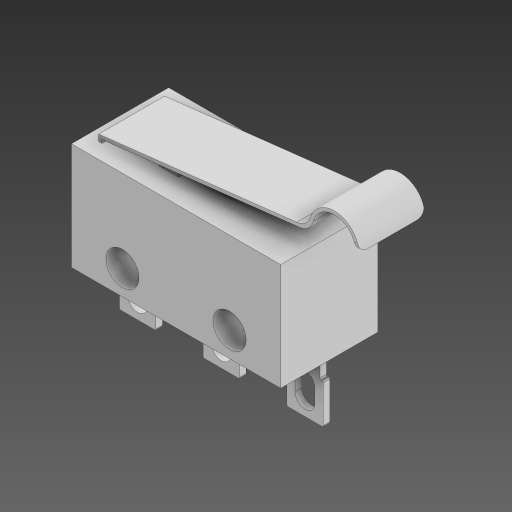
# Autodesk Inventor part: SS0750302F035S1A (Limit Switch)
Saved by Autodesk Inventor 2024 (Build 280153000, 153)
## iProperties
Created: 2024-02-03
Part Number: SS0750302F035S1A (Limit Switch)
Material: Generic
Document SubType Name: Modeling
Designer: david
Density: 1 g/cm^3
Appearance: Default
Author: david
Autodesk Inventor part; units mm, degrees
ref_plane "YZ Plane" through (0, 0, 0) normal (1, 0, 0) x (0, 1, 0)
ref_plane "XZ Plane" through (0, 0, 0) normal (0, 1, 0) x (-1, 0, 0)
ref_plane "XY Plane" through (0, 0, 0) normal (0, 0, 1) x (1, 0, 0)
sketch "Sketch1" plane through (0, 0, 0) normal (0, 0, 1) x (1, 0, 0)
  line L0 (-6.35, -3.25) -> (6.35, -3.25)
  line L1 (6.35, -3.25) -> (6.35, 3.25)
  line L2 (6.35, 3.25) -> (-6.35, 3.25)
  line L3 (-6.35, 3.25) -> (-6.35, -3.25)
  line L4 (-6.35, -3.25) -> (6.35, 3.25) construction
  line L5 (6.35, -3.25) -> (-6.35, 3.25) construction
  circle A0 centre (-3.25, -1.75) radius 1
  circle A1 centre (3.25, -1.75) radius 1
  point P0 (0, 0)
  dimension "d0" = 12.7
  dimension "d1" = 6.5
  dimension "d2" = 2
  dimension "d3" = 2
  dimension "d4" = 1.5
  dimension "d5" = 3.25
  dimension "d6" = 6.5
  constraints: 12 end point, 2 centre point, 2 midpoint, 2 parallel, 1 horizontal, 1 horizontal alignment, 1 perpendicular
  measures "d0" distance of L1.end L2.end
  measures "d1" distance of L2.end L0.start
  measures "d2" diameter of A0
  measures "d3" diameter of A1
  measures "d4" distance from line of L0 A0.centre
  measures "d5" horizontal distance of point (0, 0) A0.centre
  measures "d6" distance of A1.centre A0.centre
extrude "Extrusion1" add sketch "Sketch1" along normal blind 5.9
ref_plane "Work Plane1" through (0, 0, 2.95) normal (0, 0, 1) x (1, 0, 0)
sketch "Sketch2" plane through (0, 0, 2.95) normal (0, 0, 1) x (1, 0, 0)
  line L0 (-3.98, -4.35) -> (-3.98, -6.75)
  line L1 (-3.98, -6.75) -> (-6.18, -6.75)
  line L2 (-6.18, -6.75) -> (-6.18, -4.35)
  line L3 (-5.08, -4.95) -> (-5.08, -5.75) construction
  line L4 (-5.68, -4.95) -> (-5.68, -5.75)
  line L5 (-4.48, -5.75) -> (-4.48, -4.95)
  arc A0 (-4.48, -4.95) -> (-5.68, -4.95) centre (-5.08, -4.95) ccw
  arc A1 (-5.68, -5.75) -> (-4.48, -5.75) centre (-5.08, -5.75) ccw
  line L6 (-5.98, -3.25) -> (-4.18, -3.25)
  line L7 (-4.18, -3.25) -> (-4.18, -4.35)
  line L8 (-5.98, -4.35) -> (-5.98, -3.25)
  line L9 (-5.98, -4.35) -> (-6.18, -4.35)
  line L10 (-4.18, -4.35) -> (-3.98, -4.35)
  line L11 (-6.35, -3.25) -> (6.35, -3.25) projected
  point P0 (0, 0)
  point P1 (-5.08, -6.75)
  point P2 (-5.08, -5.35)
  point P3 (-5.08, -3.25)
  point P4 (-4.08, -4.35)
  dimension "d13" = 2.2
  dimension "d21" = 0.8
  dimension "d22" = 0.6
  dimension "d23" = 1
  dimension "d24" = 1.8
  dimension "d27" = 5.08
  dimension "d28" = 1.1
  dimension "d29" = 3.5
  constraints: 24 end point, 4 midpoint, 4 perpendicular, 4 point on circle, 4 tangent, 3 parallel, 2 centre point, 2 horizontal, 2 point on line, 2 vertical alignment, 1 vertical
  measures "d13" distance of L0.end L1.end
  measures "d21" distance of L3.end L3.start
  measures "d22" radius of A1
  measures "d23" distance of point (-5.08, -6.75) L3.end
  measures "d24" distance of L7.end L8.start
  measures "d27" horizontal distance of point (-5.08, -3.25) point (0, 0)
  measures "d28" distance from line of L11 point (-4.08, -4.35)
  measures "d29" distance between parallel lines of L1 L11
extrude "Extrusion2" add sketch "Sketch2" along normal mid plane 0.4
sketch "Sketch3" plane through (0, 0, 2.95) normal (0, 0, 1) x (1, 0, 0)
  line L0 (6.35, 3.25) -> (-6.35, 3.25) projected
  circle A0 centre (-1.95, 3.25) radius 0.6
  circle A1 centre (3.25, -1.75) radius 1 projected
  point P0 (0, 0)
  dimension "d17" = 1.2
  dimension "d18" = 5.2
  constraints: 1 centre point, 1 point on line
  measures "d17" diameter of A0
  measures "d18" horizontal distance of A1.centre A0.centre
extrude "Extrusion3" add sketch "Sketch3" along normal mid plane 2.9 contours A0 L0 | L0 A0
fillet "Fillet1" radius 0.075 6 edges at (-3.98, -4.35, 2.95) (-4.18, -4.35, 2.95) (-5.98, -4.35, 2.95) (-6.18, -4.35, 2.95) (-6.18, -6.75, 2.95) (-3.98, -6.75, 2.95)
pattern_linear "Rectangular Pattern1" count 3 spacing 5.08 along (1, 0, 0) of "Fillet1", "Extrusion2"
sketch "Sketch4" plane through (0, 0, 2.95) normal (0, 0, 1) x (1, 0, 0)
  line L0 (-6.35, 3.25) -> (-6.35, -3.25) projected
  line L1 (-6.35, -3.25) -> (6.35, -3.25) projected
  line L2 (6.35, 3.25) -> (-6.35, 3.25) projected
  circle A0 centre (8.65, 5.25) radius 1.5
  arc A1 (-1.35, 3.25) -> (-2.55, 3.25) centre (-1.95, 3.25) ccw projected
  line L3 (7.1893, 4.9089) -> (-5.45, 3.45)
  line L4 (-5.45, 3.25) -> (-5.45, 3.45)
  line L5 (-5.65, 3.25) -> (-5.65, 3.6282)
  line L6 (-5.65, 3.25) -> (-5.45, 3.25)
  line L7 (7.1569, 5.1065) -> (-5.65, 3.6282)
  circle A2 centre (8.65, 5.25) radius 1.3
  line L8 (7.1893, 4.9089) -> (7.3895, 4.932)
  line L9 (7.3895, 4.932) -> (10.15, 5.2506)
  line L10 (7.3895, 4.932) -> (10.15, 5.2506)
  line L11 (7.1569, 5.1065) -> (10.1366, 5.4504)
  point P0 (0, 0)
  point P1 (8.65, 6.75)
  point P2 (-5.55, 3.25)
  point P3 (-5.65, 3.4391)
  point P4 (-5.45, 3.35)
  point P5 (9.9498, 5.2275)
  dimension "d43" = 15
  dimension "d44" = 10
  dimension "d45" = 0.2
  dimension "d47" = 0.8
  dimension "d49" = 3
  dimension "d50" = 0.2
  dimension "d51" = 0.2
  dimension "d52" = 0.2
  constraints: 18 end point, 8 point on circle, 3 midpoint, 2 centre point, 2 parallel, 2 point on line, 2 vertical, 1 coincident, 1 collinear, 1 tangent, 1 vertical alignment
  measures "d43" distance from line of A0.start L0
  measures "d44" distance from line of L1 A0.start
  measures "d45" distance of L4.start L3.end
  measures "d47" distance from line of L0 point (-5.55, 3.25)
  measures "d49" diameter of A0
  measures "d50" distance between parallel lines of L5 L4
  measures "d51" distance between parallel lines of L3 L7
  measures "d52" radial gap between concentric circles of A0 A2
extrude "Extrusion4" add sketch "Sketch4" along normal mid plane 4 contours L3 L4 L2 L5 L7 A0 | A0 L11 A2 L8 | A0 L11 A2 | L9 A2 L11 A0
fillet "Fillet2" radius 1 2 edges at (7.3895, 4.932, 2.95) (7.1569, 5.1065, 2.95)
fillet "Fillet3" radius 0.5 2 edges at (10.0499, 5.2391, 4.95) (10.0499, 5.2391, 0.95)
equation "\"d3\" = d2"
body "Solid1"
